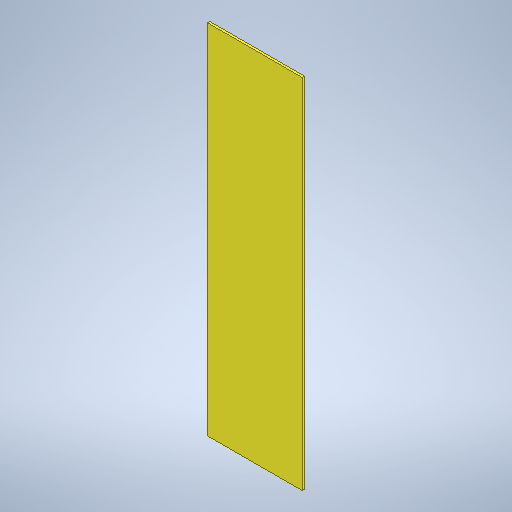
# Autodesk Inventor part: DensGlass_With_Dimensions_25.5_x_96_Inches
Saved by Autodesk Inventor 2025 (Build 290162010, 162A)
## iProperties
Created: 2024-09-16
Part Number: DensGlass_With_Dimensions_25.5_x_96_Inches
Material: Wood (Birch)
Document SubType Name: Modeling
Designer: Tom
Density: 0.55 g/cm^3
Appearance: Canary
Author: Tom
Autodesk Inventor part; units mm, degrees
ref_plane "YZ Plane" through (0, 0, 0) normal (1, 0, 0) x (0, 1, 0)
ref_plane "XZ Plane" through (0, 0, 0) normal (0, 1, 0) x (-1, 0, 0)
ref_plane "XY Plane" through (0, 0, 0) normal (0, 0, 1) x (1, 0, 0)
sketch "Sketch1" plane through (0, 0, 0) normal (0, 0, 1) x (1, 0, 0)
  line L0 (0, 0) -> (647.7, 0)
  line L1 (647.7, 0) -> (647.7, 2438.4)
  line L2 (647.7, 2438.4) -> (0, 2438.4)
  line L3 (0, 2438.4) -> (0, 0)
  dimension "d2" = 2438.4
  dimension "d3" = 647.7
  constraints: 8 end point, 2 parallel, 1 horizontal, 1 perpendicular
  measures "d2" distance of L2.end L0.start
  measures "d3" distance of L0.start L0.end
extrude "Extrusion1" add sketch "Sketch1" along normal blind 15.875
body "Solid1"
